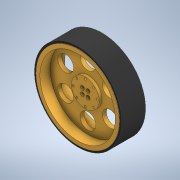
# Autodesk Inventor part: Main Wheel
Saved by Autodesk Inventor 2022 (Build 260153000, 153)
## iProperties
Created: 2022-02-10
Part Number: Main Wheel
Material: Generic
Document SubType Name: Modeling
Designer: Vedic
Density: 1 g/cm^3
Appearance: Default
Author: Vedic
Autodesk Inventor part; units mm, degrees
ref_plane "YZ Plane" through (0, 0, 0) normal (1, 0, 0) x (0, 1, 0)
sketch "Sketch1" plane through (0, 0, 0) normal (0, 0, 1) x (1, 0, 0)
  circle A0 centre (0, 0) radius 139.7
  circle A1 centre (0, 0) radius 133.35
  dimension "d0" = 279.4
  dimension "d1" = 266.7
  constraints: 2 centre point, 2 coincident
  measures "d0" diameter of A0
  measures "d1" diameter of A1
extrude "Extrusion1" add sketch "Sketch1" along normal blind 76.2
ref_plane "Work Plane1" through (0, 0, 38.1) normal (0, 0, 1) x (1, 0, 0)
sketch "Sketch2" plane through (0, 0, 38.1) normal (0, 0, 1) x (1, 0, 0)
  circle A0 centre (0, 0) radius 133.35
  circle A1 centre (0, 0) radius 120.65
  dimension "d5" = 241.3
  constraints: 2 centre point, 2 coincident
  measures "d5" diameter of A1
extrude "Extrusion2" add sketch "Sketch2" along normal mid plane 79.375
ref_plane "Work Plane2" through (0, 0, 44.45) normal (0, 0, 1) x (1, 0, 0)
sketch "Sketch3" plane through (0, 0, 44.45) normal (0, 0, 1) x (1, 0, 0)
  circle A0 centre (0, 0) radius 120.65
  circle A1 centre (0, 82.55) radius 25.4
  line L0 (0, 82.55) -> (0, 0) construction
  circle A2 centre (-71.4904, 41.275) radius 25.4
  line L1 (-71.4904, 41.275) -> (0, 0) construction
  circle A3 centre (-71.4904, -41.275) radius 25.4
  line L2 (-71.4904, -41.275) -> (0, 0) construction
  circle A4 centre (0, -82.55) radius 25.4
  line L3 (0, -82.55) -> (0, 0) construction
  circle A5 centre (71.4904, -41.275) radius 25.4
  line L4 (71.4904, -41.275) -> (0, 0) construction
  circle A6 centre (71.4904, 41.275) radius 25.4
  line L5 (71.4904, 41.275) -> (0, 0) construction
  dimension "d11" = 241.3
  dimension "d12" = 50.8
  dimension "d13" = 82.55
  dimension "d16" = 360
  constraints: 12 end point, 7 centre point, 1 coincident, 1 vertical, 25 other
  measures "d11" diameter of A0
  measures "d12" diameter of A1
  measures "d13" distance of point (0, 0) L0.start
extrude "Extrusion3" add sketch "Sketch3" against normal blind 12.7
sketch "Sketch4" plane through (0, 0, 44.45) normal (0, 0, 1) x (1, 0, 0)
  circle A0 centre (0, 0) radius 44.45
  dimension "d20" = 88.9
  constraints: 1 centre point, 1 coincident
  measures "d20" diameter of A0
extrude "Extrusion4" add sketch "Sketch4" along normal blind 8.4667
sketch "Sketch6" plane through (0, 0, 31.75) normal (0, 0, -1) x (-1, 0, 0)
  circle A0 centre (0, 0) radius 44.45
  constraints: 1 centre point, 1 coincident
extrude "Extrusion5" add sketch "Sketch6" along normal blind 0.7937
sketch "Sketch5" plane through (0, 0, 52.9167) normal (0, 0, 1) x (1, 0, 0)
  circle A0 centre (-38.1, 0) radius 3.175
  circle A1 centre (38.1, 0) radius 3.175
  circle A2 centre (0, 38.1) radius 3.175
  circle A3 centre (0, -38.1) radius 3.175
  circle A4 centre (-26.9408, 26.9408) radius 3.175
  circle A5 centre (26.9408, 26.9408) radius 3.175
  circle A6 centre (26.9408, -26.9408) radius 3.175
  circle A7 centre (-26.9408, -26.9408) radius 3.175
  line L0 (-38.1, 0) -> (0, 0) construction
  line L1 (0, 0) -> (-26.9408, 26.9408) construction
  line L2 (0, 38.1) -> (0, 0) construction
  line L3 (26.9408, 26.9408) -> (0, 0) construction
  line L4 (38.1, 0) -> (0, 0) construction
  line L5 (26.9408, -26.9408) -> (0, 0) construction
  line L6 (0, -38.1) -> (0, 0) construction
  line L7 (-26.9408, -26.9408) -> (0, 0) construction
  line L8 (-8.9803, 8.9803) -> (8.9803, 8.9803) construction
  line L9 (8.9803, 8.9803) -> (8.9803, -8.9803) construction
  line L10 (8.9803, -8.9803) -> (-8.9803, -8.9803) construction
  line L11 (-8.9803, -8.9803) -> (-8.9803, 8.9803) construction
  circle A8 centre (-8.9803, 8.9803) radius 6.35
  circle A9 centre (8.9803, 8.9803) radius 6.35
  circle A10 centre (8.9803, -8.9803) radius 6.35
  circle A11 centre (-8.9803, -8.9803) radius 6.35
  dimension "d23" = 45
  dimension "d24" = 6.35
  dimension "d25" = 38.1
  dimension "d26" = 12.7
  dimension "d27" = 12.7
  constraints: 24 end point, 12 centre point, 10 equal radius, 7 equal length, 7 perpendicular, 4 coincident, 3 point on line, 2 horizontal, 2 parallel
  measures "d23" angle of L2 L1
  measures "d24" diameter of A0
  measures "d25" distance of L0.end L0.start
  measures "d26" distance of L8.start L0.end
  measures "d27" diameter of A8
extrude "Extrusion6" cut sketch "Sketch5" against normal blind 8.4667
sketch "Sketch7" plane through (0, 0, 30.9563) normal (0, 0, -1) x (-1, 0, 0)
  circle A0 centre (0, 0) radius 25.4
  dimension "d32" = 50.8
  constraints: 1 centre point, 1 coincident
  measures "d32" diameter of A0
extrude "Extrusion7" cut sketch "Sketch7" against normal blind 13.4938
body "Solid1"
